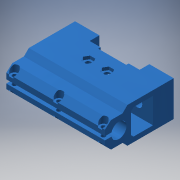
# Autodesk Inventor part: XEndBushingRight
Saved by Autodesk Inventor 2016 (Build 200138000, 138)
## iProperties
Category: Print
Created: 2014-08-15
Part Number: XEndBushingRight
Material: ABS Plastic
Document SubType Name: Modeling
Designer: t_clevj
Density: 1.06 g/cm^3
Appearance: Cyan
Mass: 65.3147 g
Surface Area: 256.51 cm^2
Volume: 61.6176 cm^3
Vendor: Jack
Author: Jack
Title: X End Right
Autodesk Inventor part; units mm, degrees
ref_plane "YZ Plane" through (0, 0, 0) normal (1, 0, 0) x (0, 1, 0)
ref_plane "XZ Plane" through (0, 0, 0) normal (0, 1, 0) x (-1, 0, 0)
ref_plane "XY Plane" through (0, 0, 0) normal (0, 0, 1) x (1, 0, 0)
sketch "Sketch1" plane through (0, 0, 0) normal (1, 0, 0) x (0, 1, 0)
  arc A0 (-6.0673, -1.5) -> (-6.0673, 1.5) centre (0, 0) ccw
  line L0 (-11.5, 1.5) -> (-11.5, 12.5)
  line L1 (-11.5, 12.5) -> (35, 12.5)
  line L2 (-11.5, -1.5) -> (-11.5, -12.5)
  line L3 (-11.5, -12.5) -> (35, -12.5)
  line L4 (-11.5, 1.5) -> (-6.0673, 1.5)
  line L5 (-11.5, -1.5) -> (-6.0673, -1.5)
  line L6 (35, 12.5) -> (35, -12.5)
  dimension "d0" = 12.5
  dimension "d1" = 1.5
  dimension "d2" = 1.5
  dimension "d3" = 11.5
  dimension "d4" = 12.5
  dimension "d5" = 12.5
  dimension "d140" = 35
  constraints: 14 end point, 3 vertical, 2 horizontal, 2 point on circle, 2 vertical alignment, 1 centre point, 1 coincident, 1 parallel, 1 perpendicular
  measures "d0" diameter of A0
  measures "d1" vertical distance of point (0, 0) L2.start
  measures "d2" vertical distance of point (0, 0) L0.start
  measures "d3" distance from line of point (0, 0) L0
  measures "d4" distance from line of point (0, 0) L1
  measures "d5" distance from line of L3 point (0, 0)
  measures "d140" distance from line of L6 point (0, 0)
extrude "MainBlock" add sketch "Sketch1" along normal blind 81
chamfer "BearingHolderChamfer" distance 5 angle 45 2 edges at (40.5, -11.5, 12.5) (40.5, -11.5, -12.5)
sketch "Sketch2" plane through (0, 35, 12.5) normal (0, 0, 1) x (1, 0, 0)
  line L0 (81, -46.5) -> (81, -41.5) projected
  line L1 (81, -41.5) -> (0, -41.5) projected
  line L2 (0, -41.5) -> (0, -46.5) projected
  line L3 (0, -46.5) -> (81, -46.5) projected
  line L4 (81, 0) -> (81, -41.5) projected
  point P0 (0, -35)
  point P1 (4, -43.75)
  point P2 (77, -43.75)
  point P3 (40.5, -43.75)
  dimension "d17" = 2.75
  dimension "d18" = 4
  dimension "d19" = 4
  dimension "d163" = 40.5
  constraints: 2 horizontal alignment
  measures "d17" distance from line of L3 point (77, -43.75)
  measures "d18" distance from line of L0 point (77, -43.75)
  measures "d19" distance from line of L2 point (4, -43.75)
  measures "d163" distance from line of L4 point (40.5, -43.75)
hole "BearingHolderClamp" at (4, -8.75, 12.5) at (77, -8.75, 12.5) at (40.5, -8.75, 12.5) direction (0, 0, -1) diameter 3.5 depth 25 tip angle 118 counterbore diameter 6.5 counterbore depth 7.75
sketch "Sketch3" plane through (81, 35, -12.5) normal (0, 0, -1) x (-1, 0, 0)
  circle A0 centre (77, -43.75) radius 1.75 projected
  circle A1 centre (77, -43.75) radius 1.75 projected
  circle A2 centre (4, -43.75) radius 1.75 projected
  circle A3 centre (4, -43.75) radius 1.75 projected
  line L0 (7.3486, -43.75) -> (5.6743, -46.65)
  line L1 (5.6743, -46.65) -> (2.3257, -46.65)
  line L2 (2.3257, -46.65) -> (0.6514, -43.75)
  line L3 (0.6514, -43.75) -> (2.3257, -40.85)
  line L4 (2.3257, -40.85) -> (5.6743, -40.85)
  line L5 (5.6743, -40.85) -> (7.3486, -43.75)
  line L6 (80.3486, -43.75) -> (78.6743, -46.65)
  line L7 (78.6743, -46.65) -> (75.3257, -46.65)
  line L8 (75.3257, -46.65) -> (73.6514, -43.75)
  line L9 (73.6514, -43.75) -> (75.3257, -40.85)
  line L10 (75.3257, -40.85) -> (78.6743, -40.85)
  line L11 (78.6743, -40.85) -> (80.3486, -43.75)
  circle A4 centre (40.5, -43.75) radius 1.75 projected
  line L12 (43.8486, -43.75) -> (42.1743, -46.65)
  line L13 (42.1743, -46.65) -> (38.8257, -46.65)
  line L14 (38.8257, -46.65) -> (37.1514, -43.75)
  line L15 (37.1514, -43.75) -> (38.8257, -40.85)
  line L16 (38.8257, -40.85) -> (42.1743, -40.85)
  line L17 (42.1743, -40.85) -> (43.8486, -43.75)
  point P0 (81, -35)
  dimension "d27" = 5.8
  dimension "d28" = 5.8
  constraints: 36 end point, 3 coincident, 2 horizontal, 1 collinear, 1 horizontal alignment, 39 other
  measures "d27" distance between parallel lines of L1 L4
  measures "d28" distance between parallel lines of L7 L10
extrude "BearingHolderNutTrap" cut sketch "Sketch3" against normal blind 7.75
sketch "Sketch4" plane through (0, 0, 0) normal (-1, 0, 0) x (0, 0, 1)
  arc A0 (1.5, -6.0673) -> (-1.5, -6.0673) centre (0, 0) ccw projected
  line L0 (-12.5, 35) -> (-12.5, -6.5) projected
  line L1 (10.5, 10) -> (-10.5, 10)
  line L2 (-10.5, 10) -> (-10.5, 28)
  line L3 (-10.5, 28) -> (10.5, 28)
  line L4 (10.5, 28) -> (10.5, 10)
  dimension "d31" = 18
  dimension "d32" = 21
  dimension "d33" = 10
  dimension "d34" = 2
  constraints: 8 end point, 2 parallel, 1 horizontal, 1 perpendicular
  measures "d31" distance of L1.end L2.end
  measures "d32" distance of L1.start L1.end
  measures "d33" distance from line of A0.centre L1
  measures "d34" distance between parallel lines of L0 L2
extrude "BeltCutoutY" cut sketch "Sketch4" against normal up to surface (81 mm away)
sketch "Sketch5" plane through (0, 35, 12.5) normal (0, 1, 0) x (1, 0, 0)
  line L0 (81, 25) -> (81, 0) projected
  line L1 (0, 25) -> (81, 25) projected
  line L2 (29, 2) -> (52, 2)
  line L3 (52, 2) -> (52, 23)
  line L4 (52, 23) -> (29, 23)
  line L5 (29, 23) -> (29, 2)
  point P0 (0, 12.5)
  dimension "d37" = 21
  dimension "d38" = 23
  dimension "d39" = 2
  dimension "d40" = 29
  constraints: 8 end point, 2 parallel, 1 horizontal, 1 perpendicular
  measures "d37" distance of L4.end L2.start
  measures "d38" distance of L2.start L2.end
  measures "d39" distance between parallel lines of L1 L4
  measures "d40" distance between parallel lines of L0 L3
extrude "BeltCutoutX" cut sketch "Sketch5" against normal up to surface (7 mm away)
sketch "Sketch6" plane through (81, 35, -12.5) normal (0, 0, -1) x (-1, 0, 0)
  line L0 (81, 0) -> (81, -41.5) projected
  line L1 (81, 0) -> (0, 0) projected
  line L2 (0, -41.5) -> (0, 0) projected
  line L3 (0, -28) -> (81, -28)
  point P0 (81, -35)
  dimension "d43" = 28
  constraints: 2 end point, 2 point on line, 1 perpendicular
  measures "d43" distance between parallel lines of L1 L3
extrude "BoltPadUpper" add sketch "Sketch6" along normal blind 2
sketch "Sketch7" plane through (0, 35, 12.5) normal (0, 0, 1) x (1, 0, 0)
  line L0 (81, 0) -> (81, -41.5) projected
  line L1 (0, 0) -> (81, 0) projected
  line L2 (0, -41.5) -> (0, 0) projected
  line L3 (0, -28) -> (0, 0) projected
  line L4 (0, -28) -> (81, -28)
  line L5 (81, 0) -> (81, -28) projected
  point P0 (0, -35)
  dimension "d46" = 28
  constraints: 2 end point, 2 point on line, 1 perpendicular
  measures "d46" distance between parallel lines of L1 L4
extrude "BoltPadLower" add sketch "Sketch7" along normal blind 2
chamfer "BoltPadChamfer" distance 2 angle 45 2 edges at (40.5, 7, 12.5) (40.5, 7, -12.5)
sketch "Sketch8" plane through (81, 35, -14.5) normal (0, 0, -1) x (-1, 0, 0)
  line L0 (81, 0) -> (0, 0) projected
  line L1 (0, 0) -> (0, -28) projected
  point P0 (81, -35)
  point P1 (32.75, -12)
  point P2 (48.25, -12)
  dimension "d54" = 12
  dimension "d116" = 15.5
  dimension "d117" = 32.75
  constraints: 1 horizontal alignment
  measures "d54" distance from line of L0 point (48.25, -12)
  measures "d116" distance of point (48.25, -12) point (32.75, -12)
  measures "d117" distance from line of L1 point (32.75, -12)
hole "BearingBoltHoles" at (48.25, 23, -14.5) at (32.75, 23, -14.5) direction (0, 0, 1) diameter 4.5 end up to face face through (27, 16.3333, 14.5) facing (0, 0, 1) counterbore diameter 8 counterbore depth 1.5
chamfer "BearingCutoutYChamfer" distance 2 angle 45 2 edges at (40.5, 10, 10.5) (40.5, 10, -10.5)
sketch "Sketch9" plane through (52, 35, 10.5) normal (0, 0, -1) x (-1, 0, 0)
  line L0 (52, -7) -> (23, -7) projected
  line L1 (23, 0) -> (23, -7) projected
  line L2 (0, 0) -> (0, -7) projected
  line L3 (0, -7) -> (-29, -7) projected
  circle A0 centre (19.25, -12) radius 2.25 projected
  circle A1 centre (3.75, -12) radius 2.25 projected
  arc A2 (0, -1.6589) -> (-6.048, -7) centre (3.75, -12) ccw
  arc A3 (29.048, -7) -> (23, -1.6589) centre (19.25, -12) ccw
  line L4 (0, -1.6589) -> (0, -7)
  line L5 (0, -7) -> (-6.048, -7)
  line L6 (23, -1.6589) -> (23, -7)
  line L7 (23, -7) -> (29.048, -7)
  point P0 (52, -35)
  dimension "d67" = 11
  dimension "d68" = 11
  constraints: 8 end point, 4 collinear, 4 point on circle, 4 point on line, 2 centre point, 2 coincident
  measures "d67" radius of A3
  measures "d68" radius of A2
sketch "Sketch10" plane through (0, 35, 14.5) normal (0, 0, 1) x (1, 0, 0)
  circle A0 centre (48.25, -12) radius 2.25 projected
  circle A1 centre (32.75, -12) radius 2.25 projected
  line L0 (37.0224, -12) -> (34.8862, -15.7)
  line L1 (34.8862, -15.7) -> (30.6138, -15.7)
  line L2 (30.6138, -15.7) -> (28.4776, -12)
  line L3 (28.4776, -12) -> (30.6138, -8.3)
  line L4 (30.6138, -8.3) -> (34.8862, -8.3)
  line L5 (34.8862, -8.3) -> (37.0224, -12)
  line L6 (52.5224, -12) -> (50.3862, -15.7)
  line L7 (50.3862, -15.7) -> (46.1138, -15.7)
  line L8 (46.1138, -15.7) -> (43.9776, -12)
  line L9 (43.9776, -12) -> (46.1138, -8.3)
  line L10 (46.1138, -8.3) -> (50.3862, -8.3)
  line L11 (50.3862, -8.3) -> (52.5224, -12)
  point P0 (0, -35)
  dimension "d71" = 7.4
  constraints: 24 end point, 2 coincident, 2 horizontal, 1 collinear, 26 other
  measures "d71" distance between parallel lines of L1 L4
extrude "BearingNutTrap" cut sketch "Sketch10" against normal blind 2.5
sketch "Sketch11" plane through (81, 35, -14.5) normal (0, 0, -1) x (-1, 0, 0)
  line L0 (81, 0) -> (0, 0) projected
  line L1 (0, 10) -> (26, 10)
  line L2 (81, 10) -> (55, 10)
  line L3 (81, 10) -> (81, 0)
  line L4 (0, 0) -> (0, 10)
  line L5 (29, 0) -> (29, 0)
  line L6 (52, 0) -> (52, 0)
  line L7 (29, 0) -> (29, 8)
  line L8 (29, 0) -> (29, -7) projected
  line L9 (52, 0) -> (52, 8)
  line L10 (55, 10) -> (52, 8)
  line L11 (26, 10) -> (29, 8)
  point P0 (81, -35)
  dimension "d74" = 26
  dimension "d75" = 26
  dimension "d80" = 10
  dimension "d93" = 8
  constraints: 20 end point, 2 horizontal, 2 perpendicular, 2 vertical, 1 collinear, 1 horizontal alignment, 1 parallel, 1 point on line
  measures "d74" distance of L1.start L1.end
  measures "d75" distance of L2.start L2.end
  measures "d80" distance of L2.start L0.start
  measures "d93" distance of L5.end L7.end
extrude "XRodHolderPad" add sketch "Sketch11" against normal up to surface (29 mm away)
sketch "Sketch15" plane through (0, 45, -14.5) normal (0, 1, 0) x (1, 0, 0)
  line L0 (55, -29) -> (81, -29) projected
  line L1 (81, 0) -> (81, -29) projected
  line L2 (55, 0) -> (81, 0) projected
  line L3 (55, 0) -> (55, -29) projected
  circle A0 centre (13, -14.5) radius 4.15
  circle A1 centre (68, -14.5) radius 4.15
  line L4 (0, 0) -> (0, -29) projected
  point P0 (0, -14.5)
  dimension "d94" = 8.3
  dimension "d95" = 8.3
  dimension "d99" = 14.5
  dimension "d137" = 13
  dimension "d154" = 13
  constraints: 2 centre point, 1 horizontal alignment
  measures "d94" diameter of A0
  measures "d95" diameter of A1
  measures "d99" distance from line of L0 A1.centre
  measures "d137" distance from line of L1 A1.centre
  measures "d154" distance from line of L4 A0.centre
extrude "XRodHole" cut sketch "Sketch15" against normal up to surface (17 mm away) contours A0 | A1
sketch "Sketch20" plane through (81, 35, -14.5) normal (0, 0, -1) x (-1, 0, 0)
  line L0 (26, 10) -> (0, 10) projected
  line L1 (0, 10) -> (0, -28) projected
  line L2 (81, -28) -> (81, 10) projected
  point P0 (81, -35)
  point P1 (68, 2)
  point P2 (13, 2)
  dimension "d122" = 8
  dimension "d123" = 13
  dimension "d124" = 13
  constraints: 1 horizontal alignment
  measures "d122" distance from line of L0 point (13, 2)
  measures "d123" distance from line of L1 point (13, 2)
  measures "d124" distance from line of L2 point (68, 2)
hole "Hole3" at (13, 37, -14.5) at (68, 37, -14.5) direction (0, 0, 1) diameter 3.5 depth 10 counterbore diameter 6.5 counterbore depth 3.7
ref_plane "Work Plane3" through (0, 35, -1) normal (0, 0, 1) x (1, 0, 0)
sketch "Sketch21" plane through (0, 35, -1) normal (0, 0, 1) x (1, 0, 0)
  circle A0 centre (13, 2) radius 1.75 projected
  circle A1 centre (68, 2) radius 1.75 projected
  line L0 (13, 5.1754) -> (15.75, 3.5877)
  line L1 (15.75, 3.5877) -> (15.75, 0.4123)
  line L2 (15.75, 0.4123) -> (13, -1.1754)
  line L3 (13, -1.1754) -> (10.25, 0.4123)
  line L4 (10.25, 0.4123) -> (10.25, 3.5877)
  line L5 (10.25, 3.5877) -> (13, 5.1754)
  line L6 (68, 5.1754) -> (70.75, 3.5877)
  line L7 (70.75, 3.5877) -> (70.75, 0.4123)
  line L8 (70.75, 0.4123) -> (68, -1.1754)
  line L9 (68, -1.1754) -> (65.25, 0.4123)
  line L10 (65.25, 0.4123) -> (65.25, 3.5877)
  line L11 (65.25, 3.5877) -> (68, 5.1754)
  point P0 (0, -35)
  dimension "d133" = 5.5
  constraints: 24 end point, 2 coincident, 2 vertical, 1 parallel, 26 other
  measures "d133" distance between parallel lines of L7 L10
extrude "Extrusion18" cut sketch "Sketch21" against normal blind 6 contours A0 | A1 | L0 L1 L2 L3 L4 L5 | L6 L7 L8 L9 L10 L11
extrude "Extrusion19" cut sketch "Sketch9" along normal up to surface (21 mm away) contours L0 L1 A3 | L2 L3 A2
sketch "Sketch26" plane through (52, 35, 10.5) normal (0, 0, -1) x (-1, 0, 0)
  circle A0 centre (3.75, -12) radius 2.25 projected
  circle A1 centre (3.75, -12) radius 4.75
  point P0 (52, -35)
  dimension "d151" = 9.5
  constraints: 1 centre point, 1 coincident
  measures "d151" diameter of A1
extrude "Extrusion24" cut sketch "Sketch26" against normal blind 0.25
sketch "Sketch27" plane through (81, 0, 0) normal (1, 0, 0) x (0, 0, -1)
  line L0 (14.5, 7) -> (12.5, 5) projected
  line L1 (-12.5, 5) -> (-14.5, 7) projected
  line L2 (-12.5, 5) -> (-12.5, -6.5) projected
  line L3 (-7.5, -11.5) -> (-12.5, -6.5) projected
  arc A0 (1.5, -6.0673) -> (-1.5, -6.0673) centre (0, 0) ccw projected
  line L4 (12.5, 5) -> (10.5, 3)
  line L5 (10.5, 3) -> (10.5, -8.5)
  line L6 (7.5, -11.5) -> (10.25, -8.75) projected
  line L7 (-12.5, 5) -> (-10.5, 3)
  line L8 (-10.5, 3) -> (-10.5, -8.5)
  line L9 (10.5, -8.5) -> (12.5, -6.5)
  line L10 (7.5, -11.5) -> (12.5, -6.5) projected
  line L11 (12.5, -6.5) -> (12.5, 5)
  dimension "d155" = 10.5
  dimension "d156" = 10.5
  constraints: 12 end point, 3 collinear, 3 vertical, 2 point on line
  measures "d155" distance from line of A0.centre L8
  measures "d156" distance from line of A0.centre L5
extrude "Extrusion27" cut sketch "Sketch27" against normal up to next
sketch "Sketch29" plane through (81, 0, 0) normal (1, 0, 0) x (0, 0, -1)
  line L0 (-10.5, 3) -> (-10.5, -8.5) projected
  line L1 (-7.5, -11.5) -> (-10.5, -8.5) projected
  line L2 (1.5, -11.5) -> (7.5, -11.5) projected
  line L3 (10.5, -8.5) -> (7.5, -11.5) projected
  line L4 (10.5, -8.5) -> (10.5, 3) projected
  line L5 (-4.75, -11.5) -> (-7.5, -11.5) projected
  line L6 (-6.125, -11.5) -> (-10.5, -6.5)
  line L7 (5.5, -11.5) -> (10.5, -6.5)
  dimension "d166" = 5
  dimension "d167" = 5
  dimension "d168" = 135
  constraints: 4 end point, 3 point on line, 1 midpoint
  measures "d166" vertical distance of L6.start L6.end
  measures "d167" horizontal distance of L7.start L7.end
  measures "d168" angle of L4 L7
extrude "Extrusion28" cut sketch "Sketch29" against normal up to surface (81 mm away)
sketch "Sketch30" plane through (55, 45, -14.5) normal (0, 1, 0) x (1, 0, 0)
  line L0 (0, -29) -> (26, -29) projected
  circle A0 centre (-42, -14.5) radius 4.15 projected
  line L1 (-55, -29) -> (-29, -29) projected
  line L2 (-29, 0) -> (-29, -29) projected
  line L3 (-55, 0) -> (-29, 0) projected
  line L4 (-55, 0) -> (-55, -29) projected
  line L5 (-26, 0) -> (-26, -29) projected
  line L6 (-3, 0) -> (-3, -29) projected
  line L7 (-3, -4) -> (-3, -25) projected
  line L8 (-3, -14.7) -> (6, -14.7)
  line L9 (6, -14.7) -> (6, -29)
  line L10 (-29, 0) -> (-29, -29) projected
  line L11 (-35, -14.7) -> (-35, -29)
  line L12 (-35, -14.7) -> (-26, -14.7)
  line L13 (-35, -29) -> (-26, -29)
  line L14 (-29, -29) -> (-26, -29) projected
  line L15 (6, -29) -> (-3, -29)
  line L16 (-3, -29) -> (0, -29) projected
  point P0 (-55, -14.5)
  dimension "d171" = 14.3
  dimension "d172" = 9
  constraints: 12 end point, 4 perpendicular, 4 point on line, 2 collinear, 2 equal length
  measures "d171" distance of L8.end L9.end
  measures "d172" distance of L8.start L8.end
extrude "Extrusion29" cut sketch "Sketch30" against normal blind 8 contours L15 L6 L8 L9 L0 | L11 L12 L2 L1 | L2 L12 L5 L13
body "Solid1"
